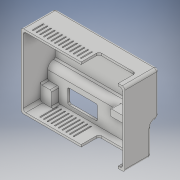
# Autodesk Inventor part: box
Saved by Autodesk Inventor 2019 (Build 230136000, 136)
## iProperties
Created: 2021-11-14
Part Number: box
Material: Generic
Document SubType Name: Modeling
Designer: Tiarnan Rice
Density: 1 g/cm^3
Appearance: Default
Author: Tiarnan Rice
Autodesk Inventor part; units mm, degrees
ref_plane "YZ Plane" through (0, 0, 0) normal (1, 0, 0) x (0, 1, 0)
sketch "Sketch1" plane through (0, 0, 0) normal (0, 0, 1) x (1, 0, 0)
  line L0 (-66.04, -45.72) -> (66.04, -45.72) construction
  line L1 (66.04, -45.72) -> (66.04, 45.72) construction
  line L2 (66.04, 45.72) -> (-66.04, 45.72) construction
  line L3 (-66.04, 45.72) -> (-66.04, -45.72) construction
  line L4 (-66.04, -45.72) -> (66.04, 45.72) construction
  line L5 (66.04, -45.72) -> (-66.04, 45.72) construction
  line L6 (-67.04, -46.72) -> (67.04, -46.72) construction
  line L7 (67.04, -46.72) -> (67.04, 46.72) construction
  line L8 (67.04, 46.72) -> (-67.04, 46.72) construction
  line L9 (-67.04, 46.72) -> (-67.04, -46.72) construction
  line L10 (-67.04, -46.72) -> (67.04, 46.72) construction
  line L11 (67.04, -46.72) -> (-67.04, 46.72) construction
  line L12 (-70.04, 49.72) -> (70.04, 49.72)
  line L13 (70.04, 49.72) -> (70.04, -49.72)
  line L14 (70.04, -49.72) -> (-70.04, -49.72)
  line L15 (-70.04, -49.72) -> (-70.04, 49.72)
  point P0 (0, 0)
  point P1 (0, 0)
  dimension "d0" = 132.08
  dimension "d1" = 91.44
  dimension "d2" = 1
  dimension "d3" = 1
  dimension "d4" = 3
  constraints: 32 end point, 6 parallel, 3 midpoint, 3 perpendicular, 2 horizontal, 1 coincident, 3 other
  measures "d0" distance of L2.end L1.end
  measures "d1" distance of L1.end L0.end
  measures "d2" distance between parallel lines of L2 L8
  measures "d3" distance between parallel lines of L7 L1
  measures "d4" distance between parallel lines of L8 L12
extrude "Extrusion1" add sketch "Sketch1" along normal blind 46
sketch "Sketch4" plane through (70.04, -49.72, 0) normal (1, 0, 0) x (0, 0, -1)
  line L0 (0, 99.44) -> (0, 0) projected
  line L1 (0, 99.44) -> (-46, 99.44) projected
  line L2 (-46, 0) -> (-46, 99.44) projected
  line L3 (0, 0) -> (-46, 0) projected
  line L4 (-10, 0) -> (-10, 35)
  arc A0 (-5, 40) -> (-10, 35) centre (-5, 35) ccw
  arc A1 (-5, 40) -> (0, 45) centre (-5, 45) ccw
  line L5 (0, 99.44) -> (0, 0) projected
  point P0 (0, 49.72)
  dimension "d14" = 10
  dimension "d15" = 35
  constraints: 4 point on circle, 3 tangent, 2 centre point, 2 end point, 2 point on line, 1 equal radius, 1 vertical, 1 vertical alignment
  measures "d14" distance between parallel lines of L0 L4
  measures "d15" distance of L4.start L4.end
extrude "Extrusion4" cut sketch "Sketch4" against normal through all contours L0 L3 L4 A0 A1
ref_plane "Work Plane1" through (67.04, -49.72, 46) normal (1, 0, 0) x (0, 0, -1)
sketch "Sketch5" plane through (67.04, -49.72, 46) normal (1, 0, 0) x (0, 0, -1)
  line L0 (36, 35) -> (36, 0) projected
  line L1 (36, 0) -> (0, 0) projected
  line L2 (0, 99.44) -> (0, 0) projected
  line L3 (46, 99.44) -> (0, 99.44) projected
  line L4 (46, 45) -> (46, 99.44) projected
  arc A0 (41, 40) -> (46, 45) centre (41, 45) ccw projected
  arc A1 (41, 40) -> (36, 35) centre (41, 35) ccw projected
  line L5 (3, 96.44) -> (3, 3)
  line L6 (3, 3) -> (33, 3)
  line L7 (33, 3) -> (33, 35)
  arc A2 (41, 43) -> (33, 35) centre (41, 35) ccw
  arc A3 (41, 43) -> (43, 45) centre (41, 45) ccw
  line L8 (43, 45) -> (43, 96.44)
  line L9 (43, 96.44) -> (3, 96.44)
  line L10 (3, 96.44) -> (0, 96.44)
  line L11 (0, 99.44) -> (0, 0) projected
  line L12 (3, 3) -> (0, 3)
  point P0 (46, 49.72)
  dimension "d20" = 3
  constraints: 14 end point, 4 point on circle, 2 centre point, 2 point on line, 1 horizontal, 1 parallel, 6 other
  measures "d20" distance between parallel lines of L3 L9
ref_plane "Work Plane2" through (-67.04, -49.72, 46) normal (-1, 0, 0) x (0, 0, 1)
extrude "Extrusion5" cut sketch "Sketch5" against normal up to surface (134.08 mm away) contours L2 L10 L5 L12 | L5 L9 L8 A3 A2 L7 L6
sketch "Sketch6" plane through (70.04, -49.72, 10) normal (0, 0, -1) x (-1, 0, 0)
  line L0 (140.08, 35) -> (140.08, 0) projected
  line L1 (0, 35) -> (140.08, 35) projected
  line L2 (0, 0) -> (0, 35) projected
  line L3 (140.08, 0) -> (0, 0) projected
  line L4 (70.08, 28) -> (110.08, 28)
  line L5 (110.08, 28) -> (110.08, 8)
  line L6 (110.08, 8) -> (70.08, 8)
  line L7 (70.08, 8) -> (70.08, 28)
  point P0 (70.04, 49.72)
  dimension "d24" = 30
  dimension "d25" = 40
  dimension "d26" = 8
  dimension "d27" = 20
  constraints: 8 end point, 2 parallel, 1 horizontal, 1 perpendicular
  measures "d24" distance between parallel lines of L0 L5
  measures "d25" distance of L4.start L4.end
  measures "d26" distance between parallel lines of L3 L6
  measures "d27" distance of L4.end L5.end
extrude "Extrusion6" cut sketch "Sketch6" against normal blind 133.5 contours L4 L5 L6 L7
fillet "Fillet4" radius 2 4 edges at (-0.04, -21.72, 11.5) (-40.04, -21.72, 11.5) (-40.04, -41.72, 11.5) (-0.04, -41.72, 11.5)
sketch "Sketch7" plane through (67.04, -46.72, 13) normal (0, 0, 1) x (1, 0, 0)
  line L0 (-67.08, 23) -> (-67.08, 7) projected
  arc A0 (-69.08, 5) -> (-67.08, 7) centre (-69.08, 7) ccw projected
  line L1 (-69.08, 5) -> (-105.08, 5) projected
  arc A1 (-107.08, 7) -> (-105.08, 5) centre (-105.08, 7) ccw projected
  line L2 (-107.08, 7) -> (-107.08, 23) projected
  arc A2 (-105.08, 25) -> (-107.08, 23) centre (-105.08, 23) ccw projected
  line L3 (-105.08, 25) -> (-69.08, 25) projected
  arc A3 (-67.08, 23) -> (-69.08, 25) centre (-69.08, 23) ccw projected
  line L4 (-134.08, 0) -> (-134.08, 32) projected
  line L5 (0, 0) -> (-134.08, 0) projected
  line L6 (0, 0) -> (0, 32) projected
  line L7 (0, 32) -> (-134.08, 32) projected
  line L8 (-134.08, 0) -> (-119.08, 0)
  line L9 (-119.08, 0) -> (-119.08, 20)
  line L10 (-119.08, 20) -> (-134.08, 20)
  line L11 (-134.08, 20) -> (-134.08, 0)
  point P0 (-67.04, 46.72)
  dimension "d31" = 15
  dimension "d32" = 20
  constraints: 8 end point, 2 parallel, 1 horizontal, 1 perpendicular
  measures "d31" distance of L10.end L9.end
  measures "d32" distance of L8.end L9.end
extrude "Extrusion7" add sketch "Sketch7" along normal blind 10 contours L4 L10 L9 L5
sketch "Sketch8" plane through (67.04, -4.72, 23) normal (0, 0, 1) x (1, 0, 0)
  line L0 (-40, -3) -> (-15, -3)
  line L1 (-15, -3) -> (-15, -12)
  line L2 (-15, -12) -> (-40, -12)
  line L3 (-40, -12) -> (-40, -3)
  line L4 (-119.08, -22) -> (-119.08, -42) projected
  line L5 (0, -42) -> (-119.08, -42) projected
  line L6 (0, -42) -> (0, -10) projected
  line L7 (0, -10) -> (-134.08, -10) projected
  line L8 (-134.08, -22) -> (-134.08, -10) projected
  line L9 (-134.08, -22) -> (-119.08, -22) projected
  line L10 (-67.08, -19) -> (-67.08, -35) projected
  arc A0 (-69.08, -37) -> (-67.08, -35) centre (-69.08, -35) ccw projected
  line L11 (-69.08, -37) -> (-105.08, -37) projected
  arc A1 (-107.08, -35) -> (-105.08, -37) centre (-105.08, -35) ccw projected
  line L12 (-107.08, -35) -> (-107.08, -19) projected
  arc A2 (-105.08, -17) -> (-107.08, -19) centre (-105.08, -19) ccw projected
  line L13 (-105.08, -17) -> (-69.08, -17) projected
  arc A3 (-67.08, -19) -> (-69.08, -17) centre (-69.08, -19) ccw projected
  point P0 (-67.04, 4.72)
  dimension "d35" = 30
  dimension "d36" = 39
  dimension "d37" = 15
  dimension "d38" = 40
  constraints: 8 end point, 2 parallel, 1 horizontal, 1 perpendicular
  measures "d35" distance between parallel lines of L2 L5
  measures "d36" distance between parallel lines of L0 L5
  measures "d37" distance between parallel lines of L6 L1
  measures "d38" distance between parallel lines of L6 L3
extrude "Extrusion8" add sketch "Sketch8" against normal up to surface (13 mm away) contours L0 L1 L7 L3 | L7 L1 L2 L3
sketch "Sketch9" plane through (67.04, -4.72, 3) normal (0, 0, 1) x (1, 0, 0)
  line L0 (-134.08, 0) -> (-134.08, 51.44) projected
  line L1 (0, 0) -> (-134.08, 0) projected
  line L2 (0, 0) -> (0, 51.44) projected
  line L3 (0, 51.44) -> (-134.08, 51.44) projected
  line L4 (-134.08, 51.44) -> (0, 51.44) projected
  line L5 (-104.08, 51.44) -> (-74.08, 51.44)
  line L6 (-74.08, 51.44) -> (-74.08, 41.44)
  line L7 (-74.08, 41.44) -> (-104.08, 41.44)
  line L8 (-104.08, 41.44) -> (-104.08, 51.44)
  point P0 (-67.04, 4.72)
  dimension "d41" = 30
  dimension "d42" = 10
  dimension "d43" = 30
  constraints: 8 end point, 2 parallel, 1 horizontal, 1 perpendicular, 1 point on line
  measures "d41" distance of L6.end L7.end
  measures "d42" distance of L5.end L6.end
  measures "d43" distance between parallel lines of L0 L8
extrude "Extrusion9" add sketch "Sketch9" along normal up to surface (20 mm away) contours L3 L6 L7 L8
fillet "Fillet5" radius 3.5 6 edges at (67.04, 46.72, 24.5) (67.04, -46.72, 28) (-70.04, -49.72, 28) (70.04, -49.72, 28) (70.04, 49.72, 23) (-70.04, 49.72, 23)
fillet "Fillet6" radius 2 10 edges at (-37.04, 46.72, 13) (-37.04, 36.72, 13) (-7.04, 36.72, 13) (-7.04, 46.72, 13) (-52.04, -26.72, 18) (-52.04, -46.72, 18) (27.04, -16.72, 18) (52.04, -16.72, 18) (52.04, -7.72, 16.5) (27.04, -7.72, 16.5)
fillet "Fillet7" radius 3.5 14 edges at (69.0149, 48.6949, 0) (70.04, 20.75, 0) (70.04, -8.2555, 1.4645) (70.04, -11.1845, 8.5355) (70.04, -30.47, 10) (69.0149, -48.6949, 10) (0, -49.72, 10) (-69.0149, -48.6949, 10) (-70.04, -30.47, 10) (-70.04, -11.1845, 8.5355) (-70.04, -8.2555, 1.4645) (-70.04, 20.75, 0) (-69.0149, 48.6949, 0) (0, 49.72, 0)
sketch "Sketch10" plane through (-66.54, -49.72, 46) normal (0, -1, 0) x (1, 0, 0)
  line L0 (116.58, -23) -> (116.58, -33) projected
  line L1 (116.58, -23) -> (95.58, -23) projected
  line L2 (95.58, -33) -> (95.58, -23) projected
  line L3 (116.58, -33) -> (95.58, -33) projected
  line L4 (77.58, 0) -> (127.58, 0)
  line L5 (127.58, 0) -> (127.58, -24)
  line L6 (127.58, -24) -> (77.58, -24)
  line L7 (77.58, -24) -> (77.58, 0)
  line L8 (133.58, 0) -> (133.58, -33) projected
  line L9 (133.58, -43) -> (133.58, 0) projected
  line L10 (133.58, -41) -> (133.58, -43) projected
  line L11 (133.58, -33) -> (133.58, -41) projected
  point P0 (66.54, -46)
  dimension "d49" = 1
  dimension "d50" = 24
  dimension "d51" = 6
  dimension "d52" = 50
  constraints: 8 end point, 2 parallel, 1 horizontal, 1 perpendicular
  measures "d49" distance between parallel lines of L6 L1
  measures "d50" distance of L4.end L5.end
  measures "d51" distance between parallel lines of L8 L5
  measures "d52" distance of L4.start L4.end
extrude "Extrusion10" cut sketch "Sketch10" against normal blind 7 contours L1 L2 L6 L7 L4 L5 L0 | L0 L6 L2 L1
fillet "Fillet8" radius 3.5 2 edges at (11.04, -48.22, 22) (61.04, -48.22, 22)
sketch "Sketch11" plane through (-66.54, -49.72, 13.5) normal (0, -1, 0) x (1, 0, 0)
  line L0 (127.58, 32.5) -> (127.58, 12) projected
  arc A0 (124.08, 8.5) -> (127.58, 12) centre (124.08, 12) ccw projected
  line L1 (124.08, 8.5) -> (81.08, 8.5) projected
  arc A1 (77.58, 12) -> (81.08, 8.5) centre (81.08, 12) ccw projected
  line L2 (77.58, 12) -> (77.58, 32.5) projected
  line L3 (0, 32.5) -> (77.58, 32.5) projected
  line L4 (0, 0) -> (0, 32.5) projected
  line L5 (133.08, 0) -> (0, 0) projected
  line L6 (133.08, 32.5) -> (133.08, 0) projected
  line L7 (18, 27.75) -> (18, 4.75) construction
  line L8 (17.25, 27.75) -> (17.25, 4.75)
  line L9 (18.75, 4.75) -> (18.75, 27.75)
  arc A2 (18.75, 27.75) -> (17.25, 27.75) centre (18, 27.75) ccw
  arc A3 (17.25, 4.75) -> (18.75, 4.75) centre (18, 4.75) ccw
  line L10 (0, 0) -> (0, 32.5) projected
  line L11 (127.58, 32.5) -> (133.08, 32.5) projected
  point P0 (66.54, -13.5)
  point P1 (18, 16.25)
  point P2 (0, 16.25)
  point P3 (0, 16.25)
  dimension "d56" = 1.5
  dimension "d57" = 23
  dimension "d58" = 18
  constraints: 8 end point, 4 point on circle, 4 tangent, 3 midpoint, 2 centre point, 2 parallel, 1 horizontal alignment
  measures "d56" diameter of A3
  measures "d57" distance of L7.start L7.end
  measures "d58" distance from line of L4 point (18, 16.25)
extrude "Extrusion11" cut sketch "Sketch11" against normal blind 7 contours A2 L9 A3 L8
pattern_linear "Rectangular Pattern1" count 10 spacing 5 along (1, 0, 0) of "Extrusion11"
sketch "Sketch12" plane through (-63.54, 46.72, 46) normal (0, -1, 0) x (1, 0, 0)
  arc A0 (15.75, -4.75) -> (14.25, -4.75) centre (15, -4.75) ccw projected
  line L0 (14.25, -27.75) -> (14.25, -4.75) projected
  line L1 (15.75, -4.75) -> (15.75, -27.75) projected
  line L2 (24.5, -23) -> (58.5, -23) projected
  line L3 (15, -4.75) -> (15, -18.75) construction
  line L4 (14.25, -4.75) -> (14.25, -18.75)
  line L5 (15.75, -18.75) -> (15.75, -4.75)
  arc A1 (15.75, -4.75) -> (14.25, -4.75) centre (15, -4.75) ccw
  arc A2 (14.25, -18.75) -> (15.75, -18.75) centre (15, -18.75) ccw
  point P0 (63.54, -46)
  point P1 (15, -11.75)
  dimension "d64" = 14
  dimension "d65" = 1.5
  constraints: 8 end point, 4 point on circle, 4 tangent, 2 centre point, 1 midpoint, 1 parallel, 1 vertical
  measures "d64" distance of L3.start L3.end
  measures "d65" distance between parallel lines of L5 L4
extrude "Extrusion12" cut sketch "Sketch12" against normal blind 7
sketch "Sketch14" plane through (-63.54, 46.72, 46) normal (0, -1, 0) x (1, 0, 0)
  arc A0 (59.25, -27.75) -> (60.75, -27.75) centre (60, -27.75) ccw projected
  line L0 (59.25, -27.75) -> (59.25, -4.75) projected
  arc A1 (60.75, -4.75) -> (59.25, -4.75) centre (60, -4.75) ccw projected
  line L1 (60.75, -4.75) -> (60.75, -27.75) projected
  arc A2 (54.25, -27.75) -> (55.75, -27.75) centre (55, -27.75) ccw projected
  line L2 (54.25, -27.75) -> (54.25, -4.75) projected
  arc A3 (55.75, -4.75) -> (54.25, -4.75) centre (55, -4.75) ccw projected
  line L3 (55.75, -4.75) -> (55.75, -27.75) projected
  arc A4 (49.25, -27.75) -> (50.75, -27.75) centre (50, -27.75) ccw projected
  line L4 (49.25, -27.75) -> (49.25, -4.75) projected
  arc A5 (50.75, -4.75) -> (49.25, -4.75) centre (50, -4.75) ccw projected
  line L5 (50.75, -4.75) -> (50.75, -27.75) projected
  arc A6 (44.25, -27.75) -> (45.75, -27.75) centre (45, -27.75) ccw projected
  line L6 (44.25, -27.75) -> (44.25, -4.75) projected
  arc A7 (45.75, -4.75) -> (44.25, -4.75) centre (45, -4.75) ccw projected
  line L7 (45.75, -4.75) -> (45.75, -27.75) projected
  arc A8 (39.25, -27.75) -> (40.75, -27.75) centre (40, -27.75) ccw projected
  line L8 (39.25, -27.75) -> (39.25, -4.75) projected
  arc A9 (40.75, -4.75) -> (39.25, -4.75) centre (40, -4.75) ccw projected
  line L9 (40.75, -4.75) -> (40.75, -27.75) projected
  arc A10 (34.25, -27.75) -> (35.75, -27.75) centre (35, -27.75) ccw projected
  line L10 (34.25, -27.75) -> (34.25, -4.75) projected
  arc A11 (35.75, -4.75) -> (34.25, -4.75) centre (35, -4.75) ccw projected
  line L11 (35.75, -4.75) -> (35.75, -27.75) projected
  arc A12 (29.25, -27.75) -> (30.75, -27.75) centre (30, -27.75) ccw projected
  line L12 (29.25, -27.75) -> (29.25, -4.75) projected
  arc A13 (30.75, -4.75) -> (29.25, -4.75) centre (30, -4.75) ccw projected
  line L13 (30.75, -4.75) -> (30.75, -27.75) projected
  arc A14 (24.25, -27.75) -> (25.75, -27.75) centre (25, -27.75) ccw projected
  line L14 (24.25, -27.75) -> (24.25, -4.75) projected
  arc A15 (25.75, -4.75) -> (24.25, -4.75) centre (25, -4.75) ccw projected
  line L15 (25.75, -4.75) -> (25.75, -27.75) projected
  arc A16 (19.25, -27.75) -> (20.75, -27.75) centre (20, -27.75) ccw projected
  line L16 (19.25, -27.75) -> (19.25, -4.75) projected
  arc A17 (20.75, -4.75) -> (19.25, -4.75) centre (20, -4.75) ccw projected
  line L17 (20.75, -4.75) -> (20.75, -27.75) projected
  arc A18 (14.25, -27.75) -> (15.75, -27.75) centre (15, -27.75) ccw projected
  line L18 (14.25, -27.75) -> (14.25, -4.75) projected
  arc A19 (15.75, -4.75) -> (14.25, -4.75) centre (15, -4.75) ccw projected
  line L19 (15.75, -4.75) -> (15.75, -27.75) projected
  line L20 (124.58, 0) -> (124.58, -20.5) projected
  arc A20 (121.08, -24) -> (124.58, -20.5) centre (121.08, -20.5) ccw projected
  line L21 (121.08, -24) -> (78.08, -24) projected
  arc A21 (74.58, -20.5) -> (78.08, -24) centre (78.08, -20.5) ccw projected
  line L22 (74.58, -20.5) -> (74.58, 0) projected
  line L23 (-3, 0) -> (74.58, 0) projected
  line L24 (-3, -32.5) -> (-3, 0) projected
  line L25 (130.08, -32.5) -> (-3, -32.5) projected
  line L26 (130.08, 0) -> (130.08, -32.5) projected
  line L27 (124.58, 0) -> (130.08, 0) projected
  line L28 (74.58, 0) -> (124.58, 0)
  point P0 (63.54, -46)
  constraints: 2 end point, 1 perpendicular
extrude "Extrusion14" cut sketch "Sketch14" against normal blind 7 contours L20 A20 L21 A21 L22 L28
pattern_linear "Rectangular Pattern3" count 12 spacing 5 along (1, 0, 0) count 3 spacing 5 along (-1, 0, 0) of "Extrusion12"
equation "\"d3\" = d2"
body "Solid1"
